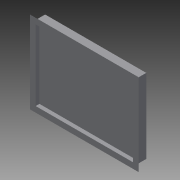
# Autodesk Inventor part: wysw trans v2
Saved by Autodesk Inventor 2014 (Build 180170000, 170)
## iProperties
Created: 2018-03-30
Part Number: wysw trans v2
Material: Generic
Document SubType Name: Modeling
Designer: HP820
Density: 1 g/cm^3
Appearance: Default
Author: HP820
Autodesk Inventor part; units mm, degrees
ref_plane "YZ Plane" through (0, 0, 0) normal (1, 0, 0) x (0, 1, 0)
ref_plane "XZ Plane" through (0, 0, 0) normal (0, 1, 0) x (-1, 0, 0)
ref_plane "XY Plane" through (0, 0, 0) normal (0, 0, 1) x (1, 0, 0)
sketch "Sketch1" plane through (0, 0, 0) normal (0, 1, 0) x (-1, 0, 0)
  line L0 (-13.3, 9.8) -> (13.3, 9.8)
  line L1 (13.3, 9.8) -> (13.3, -9.8)
  line L2 (13.3, -9.8) -> (-13.3, -9.8)
  line L3 (-13.3, -9.8) -> (-13.3, 9.8)
  line L4 (-13.3, 9.8) -> (13.3, -9.8) construction
  line L5 (13.3, 9.8) -> (-13.3, -9.8) construction
  point P0 (0, 0)
  dimension "d0" = 26.6
  dimension "d1" = 19.6
  constraints: 12 end point, 2 midpoint, 2 parallel, 1 horizontal, 1 perpendicular
  measures "d0" distance of L1.end L2.end
  measures "d1" distance of L0.end L1.end
extrude "Extrusion1" add sketch "Sketch1" along normal blind 2
sketch "Sketch2" plane through (0, 0, 0) normal (0, -1, 0) x (1, 0, 0)
  line L0 (13.3, 9.8) -> (-13.3, 9.8) projected
  line L1 (13.3, -9.8) -> (13.3, 9.8) projected
  line L2 (-14.3, -10.8) -> (14.3, -10.8)
  line L3 (14.3, -10.8) -> (14.3, 10.8)
  line L4 (14.3, 10.8) -> (-14.3, 10.8)
  line L5 (-14.3, 10.8) -> (-14.3, -10.8)
  line L6 (-14.3, -10.8) -> (14.3, 10.8) construction
  line L7 (14.3, -10.8) -> (-14.3, 10.8) construction
  point P0 (0, 0)
  dimension "d4" = 1
  dimension "d5" = 1
  constraints: 12 end point, 2 midpoint, 2 parallel, 1 horizontal, 1 perpendicular
  measures "d4" distance between parallel lines of L4 L0
  measures "d5" distance between parallel lines of L3 L1
extrude "Extrusion2" add sketch "Sketch2" along normal blind 1
chamfer "Chamfer1" distance 1 angle 45 4 edges at (0, 0, 10.8) (-14.3, 0, 0) (14.3, 0, 0) (0, 0, -10.8)
sketch "Sketch3" plane through (0, -1, 0) normal (0, -1, 0) x (1, 0, 0)
  line L0 (14.3, -10.8) -> (14.3, 10.8) projected
  line L1 (14.3, 10.8) -> (-14.3, 10.8) projected
  line L2 (-12.8, -9.3) -> (12.8, -9.3)
  line L3 (12.8, -9.3) -> (12.8, 9.3)
  line L4 (12.8, 9.3) -> (-12.8, 9.3)
  line L5 (-12.8, 9.3) -> (-12.8, -9.3)
  line L6 (-12.8, -9.3) -> (12.8, 9.3) construction
  line L7 (12.8, -9.3) -> (-12.8, 9.3) construction
  point P0 (0, 0)
  dimension "d11" = 1.5
  dimension "d12" = 1.5
  constraints: 12 end point, 2 midpoint, 2 parallel, 1 horizontal, 1 perpendicular
  measures "d11" distance between parallel lines of L1 L4
  measures "d12" distance between parallel lines of L0 L3
extrude "Extrusion3" cut sketch "Sketch3" against normal blind 1
body "Solid1"
